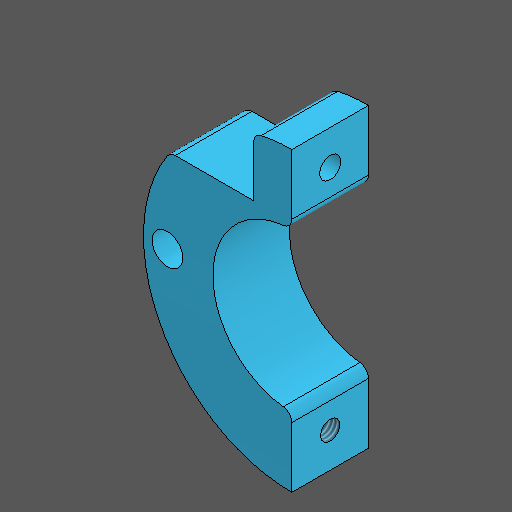
# Autodesk Inventor part: WireHolderRing-ID16.4
Saved by Autodesk Inventor 2025 (Build 290162000, 162)
## iProperties
Created: 2023-07-13
Part Number: WireHolderRing-ID16.4
Material: Stainless Steel, 440C
Document SubType Name: Modeling
Designer: kuzmin
Density: 7.75 g/cm^3
Appearance: Turquoise
Author: kuzmin
Autodesk Inventor part; units mm, degrees
ref_plane "YZ Plane" through (0, 0, 0) normal (1, 0, 0) x (0, 1, 0)
ref_plane "XZ Plane" through (0, 0, 0) normal (0, 1, 0) x (-1, 0, 0)
ref_plane "XY Plane" through (0, 0, 0) normal (0, 0, 1) x (1, 0, 0)
sketch "Sketch1" plane through (0, 0, 0) normal (0, 0, 1) x (1, 0, 0)
  circle A0 centre (0, 0) radius 8.25
  circle A1 centre (0, 0) radius 15.5
  dimension "d0" = 31
  dimension "d1" = 16.5
  constraints: 2 centre point, 2 coincident
  measures "d0" diameter of A1
  measures "d1" diameter of A0
extrude "Extrusion1" add sketch "Sketch1" along normal blind 8
sketch "Sketch2" plane through (0, 0, 8) normal (0, 0, 1) x (1, 0, 0)
  line L0 (0, -26.6625) -> (23.6951, -26.6625)
  line L1 (23.6951, -26.6625) -> (23.6951, 29.1427)
  line L2 (23.6951, 29.1427) -> (0, 29.1427)
  line L3 (0, 29.1427) -> (0, -26.6625)
  point P0 (0, 0)
  constraints: 8 end point, 2 parallel, 1 horizontal, 1 perpendicular
extrude "Extrusion2" cut sketch "Sketch2" against normal through all
sketch "Sketch3" plane through (0, 8.25, 8) normal (1, 0, 0) x (0, 0, -1)
  circle A0 centre (4, 3.625) radius 1
  line L0 (4, 3.625) -> (4, 7.25) construction
  line L1 (0, 7.25) -> (8, 7.25) projected
  line L2 (0, 0) -> (0, 7.25) projected
  point P0 (8, -8.25)
  point P1 (0, 3.625)
  dimension "d6" = 2
  constraints: 2 end point, 2 midpoint, 1 centre point, 1 horizontal alignment, 1 vertical
  measures "d6" diameter of A0
extrude "Extrusion3" cut sketch "Sketch3" against normal through all
sketch "Sketch8" plane through (0, 0, 0) normal (0, 0, -1) x (-1, 0, 0)
  line L0 (4, 8.875) -> (12.7077, 8.875)
  line L1 (12.7077, 8.875) -> (12.7077, 14.975)
  line L2 (12.7077, 14.975) -> (4, 14.975)
  line L3 (4, 14.975) -> (4, 8.875)
  arc A0 (0, -15.5) -> (0, 15.5) centre (0, 0) ccw projected
  line L4 (0, 15.5) -> (0, 8.25) projected
  point P0 (0, 11.875)
  dimension "d32" = 3
  dimension "d33" = 4
  constraints: 8 end point, 2 parallel, 2 point on circle, 1 horizontal, 1 midpoint, 1 perpendicular
  measures "d32" distance from line of L0 point (0, 11.875)
  measures "d33" distance between parallel lines of L4 L3
extrude "Extrusion7" cut sketch "Sketch8" against normal through all contours L3 A0 L0
fillet "Fillet1" radius 1 2 edges at (-12.7077, 8.875, 4) (-4, 14.975, 4)
mirror "Mirror1" about plane through (0, 0, 0) normal (0, 1, 0) of "Extrusion3"
sketch "Sketch6" plane through (0, 0, 8) normal (0, 0, 1) x (1, 0, 0)
  line L0 (0, 8.25) -> (0, 15.5) projected
  arc A0 (0, 8.25) -> (0, -8.25) centre (0, 0) ccw projected
  arc A1 (0, 15.5) -> (0, -15.5) centre (0, 0) ccw projected
  circle A2 centre (0, 0) radius 13 construction
  point P0 (-13, 0)
  point P1 (-13, 0)
  dimension "d38" = 26
  constraints: 2 coincident, 2 horizontal alignment, 2 other
hole "Hole1" at (-13, 0, 8) direction (0, 0, -1) diameter 3.2 end through all
fillet "Fillet2" radius 1 2 edges at (0, 8.25, 4) (0, -8.25, 4)
thread "Thread2" size "M2x0.4" class "6H" standard "ANSI Metric M Profile" full length
offset faces "Size2" outward -0.1 faces at (-2.6667, 11.7945, 3.0032)
equation "\"d1\" = ID"
equation "\"ID\" = 16.5"
body "Solid1"
